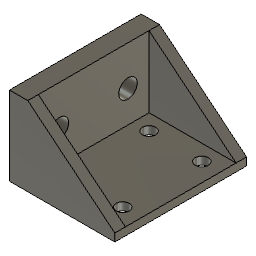
HalterungLinearantrieb (Autodesk Fusion 360 design; units mm, degrees)
part number: 2025-10-27-21-59-07-585
Autodesk Fusion 360 part; units mm, degrees
sketch "Skizze1" plane through (0, 0, 0) normal (0, 0, 1) x (1, 0, 0)
  line L0 (0, 0) -> (30, 0)
  line L1 (30, 0) -> (30, 50)
  line L2 (30, 50) -> (0, 50)
  line L3 (0, 50) -> (0, 0)
  line L4 (0, 0) -> (0, 4)
  line L5 (0, 4) -> (30, 4)
  line L6 (30, 4) -> (30, 46)
  line L7 (30, 46) -> (0, 46)
  line L8 (0, 46) -> (0, 4)
  line L9 (30, 46) -> (30, 41)
  line L10 (30, 41) -> (0, 41)
  line L11 (30, 4) -> (30, 9)
  line L12 (30, 9) -> (0, 9)
  line L13 (30, 9) -> (25, 9)
  line L14 (25, 9) -> (18, 9)
  line L15 (18, 9) -> (11, 9)
  line L16 (30, 41) -> (25, 41)
  line L17 (25, 41) -> (18, 41)
  line L18 (18, 41) -> (11, 41)
  line L19 (0, 9) -> (5, 9)
  line L20 (5, 9) -> (5, 15)
  line L21 (30, 50) -> (30, 0)
  line L22 (11, 9) -> (31, 9)
  line L23 (11, 9) -> (21, 9)
  line L24 (0, 0) -> (40, 0)
  line L25 (0, 0) -> (38, 0)
  line L26 (38, 0) -> (38, 50)
  line L27 (38, 50) -> (0, 50)
  line L28 (0, 50) -> (0, 0)
  line L29 (0, 0) -> (38, 0)
  line L30 (38, 0) -> (38, 50)
  line L31 (0, 41) -> (38, 41)
  line L32 (11, 41) -> (21, 41)
  line L33 (21, 41) -> (31, 41)
  line L34 (0, 10) -> (31, 10)
  line L35 (21, 10) -> (11, 10)
  circle A0 centre (11, 10) radius 2.5
  circle A1 centre (31, 10) radius 2.5
  circle A2 centre (11, 10) radius 5
  circle A3 centre (31, 10) radius 5
  line L36 (0, 40) -> (31, 40)
  line L37 (11, 40) -> (11, 41)
  circle A4 centre (11, 40) radius 2.5
  circle A5 centre (11, 40) radius 5
  circle A6 centre (31, 40) radius 2.5
  circle A7 centre (31, 40) radius 5
  dimension "d1" = 30
  dimension "d2" = 50
  dimension "d3" = 4
  dimension "d4" = 30
  dimension "d5" = 42
  dimension "d6" = 5
  dimension "d7" = 5
  dimension "d8" = 5
  dimension "d10" = 7
  dimension "d12" = 7
  dimension "d14" = 5
  dimension "d15" = 7
  dimension "d16" = 7
  dimension "d41" = 20
  dimension "d42" = 10
  dimension "d48" = 10
  dimension "d51" = 10
  dimension "d77" = 5
  dimension "d79" = 5
  dimension "d81" = 10
  dimension "d82" = 10
  dimension "d83" = 5
  dimension "d84" = 10
  dimension "d85" = 5
  dimension "d86" = 10
  constraint horizontal L0
  constraint vertical L1
  constraint horizontal L2
  constraint vertical L3
  constraint coincident L0.start L3.end
  constraint perpendicular L0 L4
  constraint horizontal L5
  constraint vertical L6
  constraint horizontal L7
  constraint vertical L8
  constraint perpendicular L7 L9
  constraint coincident L3 L10.end
  constraint perpendicular L5 L11
  constraint coincident L8 L12.end
  constraint perpendicular L6 L13
  constraint parallel L12 L14
  constraint parallel L12 L15
  constraint perpendicular L9 L16
  constraint parallel L10 L17
  constraint parallel L10 L18
  constraint coincident L12 L19.end
  constraint perpendicular L12 L20
  constraint vertical L21
  constraint parallel L12 L22
  constraint parallel L12 L23
  constraint coincident L24 L25.end
  constraint horizontal L27
  constraint vertical L28
  constraint horizontal L29
  constraint vertical L30
  constraint coincident L30 L31.end
  constraint perpendicular L30 L31
  constraint parallel L17 L32
  constraint parallel L31 L33
  constraint coincident L3 L34.start
  constraint perpendicular L6 L34
  constraint coincident L34 L35.start
  constraint coincident L34 L35.end
  constraint coincident L35.end A0.centre
  constraint coincident L34.end A1.centre
  constraint concentric A0 A2
  constraint coincident L8 L36.start
  constraint perpendicular L26 L36
  constraint coincident L36 L37.start
  constraint coincident L37.start A4.centre
  constraint concentric A4 A5
  constraint coincident L36.end A6.centre
  constraint concentric A6 A7
  measures "d1" distance of L0.start L0.end
  measures "d2" distance of L0.start L2.end
  measures "d3" distance of L0.start L4.end
  measures "d4" distance of L4.end L5.end
  measures "d5" distance of L4.end L7.end
  measures "d6" distance of L6.end L9.end
  measures "d7" distance of L5.end L11.end
  measures "d8" distance of L11.end L13.end
  measures "d10" distance of L13.end L14.end
  measures "d12" distance of L14.end L15.end
  measures "d14" distance of L9.end L16.end
  measures "d15" distance of L16.end L17.end
  measures "d16" distance of L17.end L18.end
  measures "d41" distance of L15.end L22.end
  measures "d42" distance of L15.end L23.end
  measures "d48" distance of L18.end L32.end
  measures "d51" distance of L32.end L33.end
  measures "d77" diameter of A0
  measures "d79" diameter of A1
  measures "d81" diameter of A2
  measures "d82" diameter of A3
  measures "d83" diameter of A4
  measures "d84" diameter of A5
  measures "d85" diameter of A6
  measures "d86" diameter of A7
extrude "Extrusion8" add sketch "Skizze1" along normal blind 3
sketch "Skizze7" plane through (0, 0, 3) normal (0, 0, 1) x (-1, 0, 0)
  line L0 (-38, 0) -> (-38, -50)
  line L1 (-38, -50) -> (0, -50)
  line L2 (0, -50) -> (0, 0)
  line L3 (0, 0) -> (-38, 0)
  line L4 (0, 0) -> (-5, 0)
  line L5 (-5, 0) -> (-5, -50)
  line L6 (-5, -50) -> (0, -50)
  line L7 (0, -50) -> (0, 0)
  constraint horizontal L4
  constraint vertical L5
  constraint horizontal L6
  constraint vertical L7
  constraint coincident L1 L5.end
  constraint coincident L2.end L3.start
extrude "Extrusion9" add sketch "Skizze7" along normal blind 27 contours L1 L2 L3 L4 L5 L6 L7
sketch "Skizze8" plane through (5, 0, 0) normal (1, 0, 0) x (0, 1, 0)
  line L0 (0, 3) -> (50, 3)
  line L1 (50, 3) -> (50, 30)
  line L2 (50, 30) -> (0, 30)
  line L3 (0, 30) -> (0, 3)
  line L4 (0, 30) -> (0, 15)
  line L5 (0, 15) -> (50, 15)
  line L6 (25, 15) -> (15, 15)
  line L7 (0, 30) -> (5, 30)
  line L8 (5, 30) -> (5, 3)
  line L9 (5, 3) -> (0, 3)
  line L10 (0, 3) -> (0, 30)
  line L11 (50, 30) -> (45, 30)
  line L12 (45, 30) -> (45, 3)
  line L13 (45, 3) -> (50, 3)
  line L14 (50, 3) -> (50, 30)
  line L15 (45, 15) -> (38, 15)
  line L16 (5, 15) -> (12, 15)
  circle A0 centre (12, 15) radius 3.5
  circle A1 centre (38, 15) radius 3.5
  dimension "d59" = 7
  dimension "d60" = 7
  dimension "d61" = 7
  dimension "d62" = 7
  constraint coincident L2.end L3.start
  constraint coincident L3 L4.end
  constraint coincident L1 L5.end
  constraint perpendicular L1 L5
  constraint midpoint L5 L6.start
  constraint perpendicular L4 L6
  constraint horizontal L7
  constraint vertical L8
  constraint horizontal L9
  constraint vertical L10
  constraint coincident L0 L8.end
  constraint horizontal L11
  constraint vertical L12
  constraint horizontal L13
  constraint vertical L14
  constraint coincident L0 L12.end
  constraint coincident L1.end L2.start
  constraint coincident L5 L15.start
  constraint coincident L12 L15.start
  constraint perpendicular L12 L15
  constraint coincident L8 L16.start
  constraint coincident L5 L16.start
  constraint perpendicular L8 L16
  constraint coincident L16.end A0.centre
  constraint coincident L15.end A1.centre
  measures "d59" distance of L15.start L15.end
  measures "d60" distance of L16.start L16.end
  measures "d61" diameter of A0
  measures "d62" diameter of A1
sketch "Skizze9" plane through (0, 0, 0) normal (0, 1, 0) x (1, 0, 0)
  line L0 (5, -30) -> (38, -3)
  line L1 (5, -30) -> (5, -3)
  line L2 (5, -3) -> (38, -3)
  constraint vertical L1
  constraint perpendicular L1 L2
extrude "Extrusion10" add sketch "Skizze9" along normal blind 5
extrude "Extrusion11" add 1 faces at (16, 5, 12) along direction (0, 1, 0) blind 5 from surface at 40
extrude "Extrusion12" cut sketch "Skizze8" against normal blind 19 contours L5 L6 L16 A0 | L5 L6 L16 A0 | L5 L15 A1 | L5 L15 A1
extrude "Extrusion13" add 1 faces at (0, 21.0929, 3.914) along direction (-1, 0, 0) blind 2
sketch "Skizze10" plane through (5, 0, 0) normal (1, 0, 0) x (0, 1, 0)
  circle A0 centre (38, 15) radius 3.5
  circle A1 centre (12, 15) radius 3.5
  line L0 (45, 3) -> (45, 30)
  line L1 (45, 30) -> (5, 30)
  line L2 (5, 30) -> (5, 3)
  line L3 (5, 3) -> (45, 3)
sketch "Skizze11" plane through (0, 0, 3) normal (0, 0, 1) x (-1, 0, 0)
  line L0 (-38, -45) -> (-5, -45)
  line L1 (-5, -45) -> (-5, -5)
  line L2 (-5, -5) -> (-38, -5)
  line L3 (-38, -5) -> (-38, -45)
  circle A0 centre (-11, -9) radius 4.55
  dimension "d72" = 9.1
  measures "d72" diameter of A0
extrude "Extrusion14" cut 1 faces at (16, 5, 12) along direction (0, -1, 0) blind 1
extrude "Extrusion15" cut 1 faces at (16, 45, 12) along direction (0, 1, 0) blind 1
extrude "Extrusion16" cut sketch "Skizze1" along normal blind 4 contours L1 L6 L11 L12 L13 L21 L22 A1 | L1 L6 L11 L21 A1 | L1 L6 L12 L13 L21 L22 L34 A1 | L1 L6 L21 L34 A1
extrude "Extrusion17" cut sketch "Skizze1" along normal blind 11 contours L1 L6 L21 L31 L33 A6 | L1 L6 L9 L21 L31 L33 A6 | L1 L6 L9 L10 L16 L21 L31 L33 A6 | L1 L6 L21 L36 A6 | L1 L6 L10 L16 L21 L31 L33 L36 A6
extrude "Extrusion18" cut sketch "Skizze1" along normal blind 5 contours L10 L31 L36 L37 A4 | L36 A4 | L10 L18 L31 L32 A4 | L10 L18 L31 L32 L36 L37 A4
extrude "Extrusion19" cut sketch "Skizze1" along normal blind 6 contours L12 L15 L22 L23 L34 L35 A0 | L12 L15 L22 L23 A0 | L34 L35 A0
